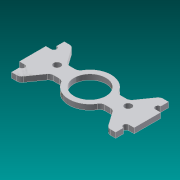
# Autodesk Inventor part: 足首_サブフレーム_1_2
Saved by Autodesk Inventor 2016 (Build 200138000, 138)
## iProperties
Created: 2016-04-30
Part Number: 足首_サブフレーム_1_2
Material: アルミニウム 2014-T4
Document SubType Name: Modeling
Designer: hiroaki
Density: 2.8 g/cm^3
Appearance: サテン
Mass: 2.26574 g
Surface Area: 12.2378 cm^2
Volume: 0.809192 cm^3
Author: hiroaki
Autodesk Inventor part; units mm, degrees
ref_plane "YZ Plane" through (0, 0, 0) normal (1, 0, 0) x (0, 1, 0)
ref_plane "XZ Plane" through (0, 0, 0) normal (0, 1, 0) x (-1, 0, 0)
ref_plane "XY Plane" through (0, 0, 0) normal (0, 0, 1) x (1, 0, 0)
sketch "スケッチ1" plane through (0, 0, 0) normal (0, 0, 1) x (1, 0, 0)
  circle A0 centre (0, 0) radius 10.5 construction
  circle A1 centre (-13.5, 1) radius 1.35
  line L0 (-13.5, 28) -> (13.5, 28) construction
  line L1 (13.5, 28) -> (13.5, 1) construction
  line L2 (13.5, 1) -> (-13.5, 1) construction
  line L3 (-13.5, 1) -> (-13.5, 28) construction
  circle A2 centre (-13.5, 28) radius 1.35
  circle A3 centre (13.5, 1) radius 1.35
  circle A4 centre (13.5, 28) radius 1.35
  line L4 (-19.75, 10) -> (-19.75, 7.1)
  line L5 (-19.75, 10) -> (19.75, 10)
  line L6 (19.75, 10) -> (19.75, 7.1)
  line L7 (-19.75, -7.1) -> (-19.75, -10)
  line L8 (-19.75, -10) -> (19.75, -10)
  line L9 (19.75, -7.1) -> (19.75, -10)
  line L10 (-19.75, 5) -> (-21.75, 5)
  line L11 (-21.75, 5) -> (-21.75, -5)
  line L12 (-21.75, -5) -> (-19.75, -5)
  arc A5 (-19.75, 5) -> (-19.75, 7.1) centre (-19.75, 6.05) ccw
  arc A6 (-19.75, -7.1) -> (-19.75, -5) centre (-19.75, -6.05) ccw
  line L13 (19.75, 5) -> (21.75, 5)
  line L14 (21.75, 5) -> (21.75, -5)
  line L15 (21.75, -5) -> (19.75, -5)
  arc A7 (19.75, 7.1) -> (19.75, 5) centre (19.75, 6.05) ccw
  line L16 (0, 28) -> (0, 0) construction
  arc A8 (19.75, -5) -> (19.75, -7.1) centre (19.75, -6.05) ccw
  line L17 (-21.75, 0) -> (21.75, 0) construction
  circle A9 centre (0, 0) radius 6.05
  point P0 (0, 10)
  dimension "d8" = 21
  dimension "d10" = 27
  dimension "d12" = 1
  dimension "d13" = 2.7
  dimension "d38" = 27
  dimension "d44" = 27
  dimension "d47" = 1.05
  dimension "d48" = 39.5
  dimension "d49" = 2
  dimension "d50" = 10
  dimension "d51" = 5
  dimension "d52" = 12.1
  constraints: 36 end point, 10 centre point, 9 perpendicular, 8 point on circle, 7 vertical alignment, 5 midpoint, 5 vertical, 4 horizontal, 4 tangent, 3 coincident, 3 equal radius, 2 parallel, 2 symmetric about line, 1 horizontal alignment, 8 other
  measures "d8" diameter of A0
  measures "d10" distance of L0.start L0.end
  measures "d12" distance from line of point (0, 0) L2
  measures "d13" diameter of A1
  measures "d38" distance of A1.centre A2.centre
  measures "d44" distance of A1.centre A3.centre
  measures "d47" radius of A5
  measures "d48" distance of L4.start L5.end
  measures "d49" distance between parallel lines of L11 L4
  measures "d50" distance between parallel lines of L12 L10
  measures "d51" distance between parallel lines of L5 L10
  measures "d52" diameter of A9
extrude "押し出し1" add sketch "スケッチ1" along normal blind 2 contours L5 L6 A7 L13 L14 L15 A8 L9 L8 L7 A6 L12 L11 L10 A5 L4
sketch "スケッチ2" plane through (0, 0, 2) normal (0, 0, 1) x (1, 0, 0)
  circle A0 centre (0, 0) radius 6.05 projected
  circle A1 centre (-13.5, 1) radius 1.35 projected
  line L0 (-19.75, -10) -> (19.75, -10) projected
  line L1 (19.75, 10) -> (-19.75, 10) projected
  line L2 (-11.8485, 3) -> (-7.4162, 3)
  arc A2 (7.4162, 3) -> (-7.4162, 3) centre (0, 0) ccw
  line L3 (7.4162, 3) -> (11.8485, 3)
  line L4 (-18.4641, 12.448) -> (18.4641, 12.448)
  line L5 (-18.4641, 12.448) -> (-11.8485, 3)
  line L6 (11.8485, 3) -> (18.4641, 12.448)
  line L7 (-11.8485, -3) -> (-7.4162, -3)
  line L8 (-11.8485, -3) -> (-24.333, -20.8295)
  line L9 (-24.333, -20.8295) -> (24.333, -20.8295)
  line L10 (11.8485, -3) -> (7.4162, -3)
  line L11 (11.8485, -3) -> (24.333, -20.8295)
  arc A3 (-7.4162, -3) -> (7.4162, -3) centre (0, 0) ccw
  line L12 (-21.75, 5) -> (-21.75, -5) projected
  line L13 (-16.75, 10) -> (-19.75, 10) construction
  line L14 (0, 0) -> (-21.75, 0) construction
  line L15 (-19.75, -10) -> (-16.75, -10) construction
  line L16 (-19.75, -10) -> (19.75, -10) construction
  line L17 (0, 0) -> (0, 10) construction
  line L18 (19.75, 10) -> (16.75, 10) construction
  line L19 (19.75, -10) -> (16.75, -10) construction
  circle A4 centre (-13.5, 1) radius 2.5 construction
  dimension "d57" = 8
  dimension "d58" = 3
  dimension "d60" = 6
  dimension "d64" = 3
  dimension "d65" = 5
  constraints: 32 end point, 8 point on line, 6 horizontal, 4 point on circle, 3 centre point, 3 coincident, 3 symmetric about line, 3 vertical alignment, 2 horizontal alignment, 2 midpoint, 1 collinear, 1 concentric, 1 tangent
  measures "d57" radius of A2
  measures "d58" distance from line of A0.centre L2
  measures "d60" distance between parallel lines of L3 L10
  measures "d64" distance of L13.start L1.end
  measures "d65" diameter of A4
extrude "押し出し2" cut sketch "スケッチ2" against normal blind 10 contours L8 L7 A3 L10 L11 L0 | L0 L11 L9 L8 | L6 L3 A2 L2 L5 L1 | L1 L5 L4 L6
fillet "フィレット1" radius 2 12 edges at (-11.8485, 3, 1) (-7.4162, 3, 1) (7.4162, 3, 1) (11.8485, -3, 1) (7.4162, -3, 1) (-7.4162, -3, 1) (-11.8485, -3, 1) (-16.75, -10, 1) (-16.75, 10, 1) (16.75, 10, 1) (16.75, -10, 1) (11.8485, 3, 1)
equation "\"d38\" = d10"
equation "\"d44\" = d10"
equation "\"d50\" = d11"
equation "\"d51\" = d28"
equation "\"d60\" = 2 * d58"
equation "\"d11\" = 10"
equation "\"d28\" = 5"
